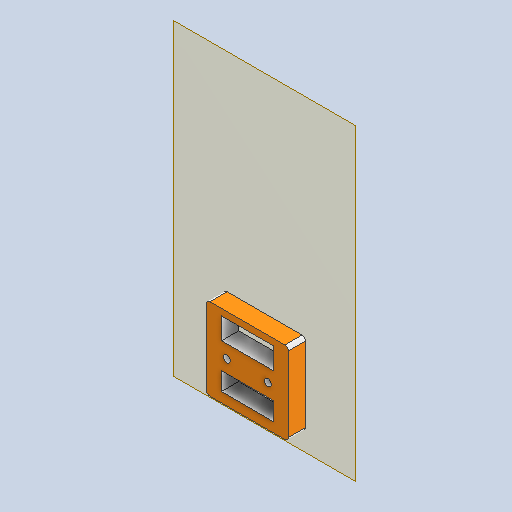
# Autodesk Inventor part: голова
Saved by Autodesk Inventor 2024.2 (Build 282272000, 272)
## iProperties
Created: 2025-10-19
Part Number: голова
Material: PA-CF
Document SubType Name: Modeling
Designer: katya_notebook
Density: 1.18 g/cm^3
Appearance: Типовые
Author: katya_notebook
Autodesk Inventor part; units mm, degrees
ref_plane "YZ Plane" through (0, 0, 0) normal (1, 0, 0) x (0, 1, 0)
ref_plane "XZ Plane" through (0, 0, 0) normal (0, 1, 0) x (-1, 0, 0)
ref_plane "XY Plane" through (0, 0, 0) normal (0, 0, 1) x (1, 0, 0)
ref_plane "РабПлоскость1" through (0, 0.0753, 0) normal (0, 0, 1) x (1, 0, 0)
sketch "Эскиз1" plane through (0, 0.0753, 0) normal (0, 0, 1) x (1, 0, 0)
  line L0 (-20, -75.0753) -> (20, -35.0753) construction
  line L1 (20, -75.0753) -> (-20, -35.0753) construction
  line L2 (51, -61.9533) -> (51, 1.0467) projected
  line L3 (-51, 1.0467) -> (-51, -61.9533) projected
  line L4 (23.7454, -78.8207) -> (-23.7454, -78.8207)
  line L5 (-23.7454, -78.8207) -> (-23.7454, -31.3299)
  line L6 (-23.7454, -31.3299) -> (23.7454, -31.3299)
  line L7 (23.7454, -31.3299) -> (23.7454, -78.8207)
  line L8 (23.7454, -78.8207) -> (-23.7454, -31.3299) construction
  line L9 (-23.7454, -78.8207) -> (23.7454, -31.3299) construction
  point P0 (0, -0.0753)
  point P1 (0, -55.0753)
  point P2 (0, -55.0753)
  dimension "d0" = 40
  dimension "d1" = 40
  dimension "d2" = 55
  dimension "d3" = 51
  constraints: 16 end point, 4 midpoint, 2 parallel, 1 horizontal, 1 perpendicular, 1 point on line
  measures "d0" distance of L1.start L0.end
  measures "d1" distance of L0.end L1.end
  measures "d2" distance of point (0, -0.075) point (0, -55.075)
  measures "d3" distance from line of point (0, -55.075) L2
extrude "Выдавливание1" add sketch "Эскиз1" along normal blind 10
fillet "Сопряжение1" radius 2 4 edges at (-23.7454, -78.7454, 5) (23.7454, -78.7454, 5) (23.7454, -31.2546, 5) (-23.7454, -31.2546, 5)
sketch "Эскиз2" plane through (0, 0.0753, 10) normal (0, 0, 1) x (1, 0, 0)
  line L0 (21.7454, -31.3299) -> (-21.7454, -31.3299) projected
  line L1 (0, -31.3299) -> (0, -78.8207)
  line L2 (-21.7454, -78.8207) -> (21.7454, -78.8207) projected
  line L3 (-23.7454, -33.3299) -> (-23.7454, -76.8207) projected
  line L4 (-23.7454, -55.0753) -> (23.7454, -55.0753)
  line L5 (23.7454, -76.8207) -> (23.7454, -33.3299) projected
  line L6 (0, -55.0753) -> (-11.8725, -55.0753)
  circle A0 centre (-11.8725, -55.0753) radius 2
  circle A1 centre (11.8725, -55.0753) radius 2
  point P0 (0, -0.0753)
  point P1 (0, -55.0753)
  dimension "d7" = 11.8725
  dimension "d8" = 4
  constraints: 6 end point, 6 midpoint, 2 centre point, 1 coincident, 1 point on line, 1 symmetric about line, 1 other
  measures "d7" distance of point (0, -55.075) L6.end
  measures "d8" diameter of A0
extrude "Выдавливание2" cut sketch "Эскиз2" against normal blind 10
sketch "Эскиз3" plane through (0, 0.0753, 10) normal (0, 0, 1) x (1, 0, 0)
  line L0 (-21.7454, -78.8207) -> (21.7454, -78.8207) projected
  line L1 (0, -78.8207) -> (0, -31.3299)
  line L2 (21.7454, -31.3299) -> (-21.7454, -31.3299) projected
  line L3 (-23.7454, -33.3299) -> (-23.7454, -76.8207) projected
  line L4 (-23.7454, -55.0753) -> (23.7454, -55.0753)
  line L5 (23.7454, -76.8207) -> (23.7454, -33.3299) projected
  line L6 (15, -75.0707) -> (-15, -75.0707)
  line L7 (-15, -75.0707) -> (-15, -62.5707)
  line L8 (-15, -62.5707) -> (15, -62.5707)
  line L9 (15, -62.5707) -> (15, -75.0707)
  line L10 (15, -75.0707) -> (-15, -62.5707) construction
  line L11 (-15, -75.0707) -> (15, -62.5707) construction
  line L12 (-21.7454, -78.8207) -> (21.7454, -78.8207) projected
  line L13 (15, -35.0799) -> (-15, -35.0799)
  line L14 (-15, -35.0799) -> (-15, -47.5799)
  line L15 (-15, -47.5799) -> (15, -47.5799)
  line L16 (15, -47.5799) -> (15, -35.0799)
  point P0 (0, -0.0753)
  point P1 (0, -68.8207)
  dimension "d11" = 30
  dimension "d12" = 12.5
  dimension "d13" = 10
  constraints: 24 end point, 7 midpoint, 4 symmetric about line, 2 parallel, 1 horizontal, 1 perpendicular, 1 point on line
  measures "d11" distance of L7.end L8.end
  measures "d12" distance of L8.end L6.start
  measures "d13" distance of point (0, -78.821) point (0, -68.821)
extrude "Выдавливание3" cut sketch "Эскиз3" against normal blind 10
sketch "Эскиз4" plane through (-15, -74.9954, 10) normal (0, 1, 0) x (1, 0, 0)
  line L0 (74.4394, -8) -> (-39.5596, -8) projected
  line L1 (30, 0) -> (0, 0) projected
  line L2 (30, 0) -> (30, 10) projected
  line L3 (0, 10) -> (30, 10) projected
  line L4 (0, 0) -> (0, 10) projected
  point P0 (15, 10)
ref_plane "РабПлоскость2" through (-14.9975, -72.9954, 9.931) normal (0.0042784, 0.9999908, 0) x (0, 0, 1)
extrude "Выдавливание4" add sketch "Эскиз4" along normal up to surface surface through (-14.9975, -72.9954, 9.931) normal (0.0042784, 0.9999908, 0)
